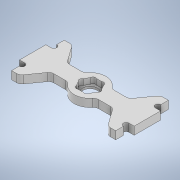
# Autodesk Inventor part: Ankle_front_frame
Saved by Autodesk Inventor 2020 (Build 240168000, 168)
## iProperties
Created: 2021-10-01
Part Number: Ankle_front_frame
Material: アルミニウム 2014-T4
Document SubType Name: Modeling
Designer: Masato Kubotera
Density: 2.8 g/cm^3
Appearance: 滑らか - 淡い灰色
Description: A2017 T3
Mass: 3.73325 g
Surface Area: 14.0657 cm^2
Volume: 1.3333 cm^3
Author: Masato Kubotera
Autodesk Inventor part; units mm, degrees
ref_plane "YZ Plane" through (0, 0, 0) normal (1, 0, 0) x (0, 1, 0)
ref_plane "XZ Plane" through (0, 0, 0) normal (0, 1, 0) x (-1, 0, 0)
ref_plane "XY Plane" through (0, 0, 0) normal (0, 0, 1) x (1, 0, 0)
sketch "スケッチ1" plane through (0, 0, 0) normal (0, 0, 1) x (1, 0, 0)
  line L0 (-19.75, 10) -> (19.75, 10) construction
  line L1 (19.75, 10) -> (19.75, -10) construction
  line L2 (19.75, -10) -> (-19.75, -10) construction
  line L3 (-19.75, -10) -> (-19.75, 10) construction
  line L4 (-19.75, 10) -> (19.75, -10) construction
  line L5 (19.75, 10) -> (-19.75, -10) construction
  line L6 (-19.75, 5) -> (-21.75, 5)
  line L7 (-21.75, 5) -> (-21.75, -5)
  line L8 (-19.75, 0) -> (19.75, 0) construction
  line L9 (0, 10) -> (0, -10) construction
  circle A0 centre (0, 0) radius 2.75
  arc A1 (-19.75, 5) -> (-19.75, 7.1) centre (-19.75, 6.05) ccw
  line L10 (-16.75, 10) -> (-11.75, 3)
  line L11 (-19.75, -5) -> (-21.75, -5)
  arc A2 (-19.75, -7.1) -> (-19.75, -5) centre (-19.75, -6.05) ccw
  line L12 (-16.75, -10) -> (-11.75, -3)
  line L13 (-19.75, 7.1) -> (-19.75, 10)
  line L14 (-16.75, 10) -> (-19.75, 10)
  line L15 (-16.75, -10) -> (-19.75, -10)
  line L16 (-19.75, -7.1) -> (-19.75, -10)
  line L17 (19.75, 5) -> (21.75, 5)
  line L18 (21.75, 5) -> (21.75, -5)
  arc A3 (19.75, 7.1) -> (19.75, 5) centre (19.75, 6.05) ccw
  line L19 (16.75, 10) -> (11.75, 3)
  line L20 (19.75, -5) -> (21.75, -5)
  arc A4 (19.75, -5) -> (19.75, -7.1) centre (19.75, -6.05) ccw
  line L21 (16.75, -10) -> (11.75, -3)
  line L22 (19.75, 7.1) -> (19.75, 10)
  line L23 (16.75, 10) -> (19.75, 10)
  line L24 (16.75, -10) -> (19.75, -10)
  line L25 (19.75, -7.1) -> (19.75, -10)
  arc A5 (5.1962, 3) -> (-5.1962, 3) centre (0, 0) ccw
  arc A6 (-5.1962, -3) -> (5.1962, -3) centre (0, 0) ccw
  line L26 (-2.0265, -3.51) -> (-2.5515, -2.6007) construction
  line L27 (-4.053, 0) -> (-3.528, 0.9093) construction
  line L28 (-2.0265, 3.51) -> (-0.9765, 3.51) construction
  line L29 (2.0265, 3.51) -> (2.5515, 2.6007) construction
  line L30 (4.053, 0) -> (3.528, -0.9093) construction
  line L31 (2.0265, -3.51) -> (0.9765, -3.51) construction
  arc A7 (-3.528, 0.9093) -> (-3.528, -0.9093) centre (-3.003, 0) ccw
  arc A8 (-2.5515, -2.6007) -> (-0.9765, -3.51) centre (-1.5015, -2.6007) ccw
  arc A9 (0.9765, -3.51) -> (2.5515, -2.6007) centre (1.5015, -2.6007) ccw
  arc A10 (3.528, -0.9093) -> (3.528, 0.9093) centre (3.003, 0) ccw
  arc A11 (2.5515, 2.6007) -> (0.9765, 3.51) centre (1.5015, 2.6007) ccw
  arc A12 (-0.9765, 3.51) -> (-2.5515, 2.6007) centre (-1.5015, 2.6007) ccw
  line L32 (-2.5515, 2.6007) -> (-2.0265, 3.51) construction
  line L33 (-3.528, 0.9093) -> (-2.5515, 2.6007)
  line L34 (-3.528, -0.9093) -> (-4.053, 0) construction
  line L35 (-2.5515, -2.6007) -> (-3.528, -0.9093)
  line L36 (-0.9765, -3.51) -> (-2.0265, -3.51) construction
  line L37 (0.9765, -3.51) -> (-0.9765, -3.51)
  line L38 (2.5515, -2.6007) -> (2.0265, -3.51) construction
  line L39 (3.528, -0.9093) -> (2.5515, -2.6007)
  line L40 (3.528, 0.9093) -> (4.053, 0) construction
  line L41 (2.5515, 2.6007) -> (3.528, 0.9093)
  line L42 (0.9765, 3.51) -> (2.0265, 3.51) construction
  line L43 (-0.9765, 3.51) -> (0.9765, 3.51)
  line L44 (-11.75, 3) -> (-5.1962, 3)
  line L45 (-5.1962, -3) -> (-11.75, -3)
  line L46 (5.1962, -3) -> (11.75, -3)
  line L47 (11.75, 3) -> (5.1962, 3)
  point P0 (0, 0)
  dimension "d0" = 39.5
  dimension "d3" = 5.5
  dimension "d4" = 2
  dimension "d5" = 10
  dimension "d6" = 1.05
  dimension "d7" = 3
  dimension "d9" = 5
  dimension "d11" = 8
  dimension "d12" = 6
  dimension "d14" = 1.05
  dimension "d17" = 360
  dimension "d19" = 7.02
  dimension "d20" = 6
  constraints: 96 end point, 25 point on circle, 21 symmetric about line, 13 centre point, 10 midpoint, 5 collinear, 5 point on line, 4 parallel, 3 horizontal, 3 perpendicular, 1 coincident, 48 other
  measures "d0" distance of L1.end L2.end
  measures "d3" diameter of A0
  measures "d4" distance of L6.start L6.end
  measures "d5" distance of L6.end L7.end
  measures "d6" radius of A1
  measures "d7" distance of L10.start L0.start
  measures "d9" vertical distance of L6.end L0.start
  measures "d11" horizontal distance of L0.start L10.end
  measures "d12" radius of A5
  measures "d14" radius of A7
  measures "d19" distance between parallel lines of L39 L33
  measures "d20" distance between parallel lines of L45 L44
extrude "押し出し1" add sketch "スケッチ1" along normal blind 3 contours A1 L13 L14 L10 L44 A5 L47 L19 L23 L22 A3 L17 L18 L20 A4 L25 L24 L21 L46 A6 L45 L12 L15 L16 A2 L11 L7 L6
extrude "押し出し2" add sketch "スケッチ1" along normal blind 0.8 contours L33 A12 L43 A11 L41 A10 L39 A9 L37 A8 L35 A7
fillet "フィレット1" radius 2 12 edges at (-11.75, 3, 1.5) (-11.75, -3, 1.5) (-16.75, 10, 1.5) (-16.75, -10, 1.5) (-5.1962, -3, 1.5) (-5.1962, 3, 1.5) (5.1962, 3, 1.5) (5.1962, -3, 1.5) (11.75, 3, 1.5) (11.75, -3, 1.5) (16.75, 10, 1.5) (16.75, -10, 1.5)
